Wood Protectors (Autodesk Fusion 360 design; units mm, degrees)
Autodesk Fusion 360 part; units mm, degrees
sketch "Sketch1" plane through (0, 0, 0) normal (0, 0, 1) x (1, 0, 0)
  circle A0 centre (-60, 0) radius 3
  circle A1 centre (-60, 0) radius 6.5
  dimension "d6" = 6
  dimension "d7" = 13
  constraint concentric A0 A1
  measures "d6" diameter of A0
  measures "d7" diameter of A1
sketch "Sketch2" plane through (0, 0, 0) normal (0, 0, 1) x (1, 0, 0)
  circle A0 centre (15.4632, 32.9185) radius 3
  circle A1 centre (9.4904, 74.3706) radius 3
  circle A2 centre (15.3555, 112.4631) radius 3
  line L0 (-7.5554, 127.9921) -> (32.4446, 127.9921)
  line L1 (32.4446, 127.9921) -> (32.4446, 17.9921)
  line L2 (32.4446, 17.9921) -> (-7.5554, 17.9921)
  line L3 (-7.5554, 17.9921) -> (-7.5554, 127.9921)
  dimension "d18" = 6
  dimension "d19" = 6
  dimension "d20" = 6
  dimension "d22" = 40
  dimension "d23" = 110
  constraint horizontal L0
  constraint vertical L1
  constraint horizontal L2
  constraint vertical L3
  measures "d18" diameter of A0
  measures "d19" diameter of A1
  measures "d20" diameter of A2
  measures "d22" distance of L1 L3
  measures "d23" distance of L0 L2
extrude "Extrude1" add sketch "Sketch1" along normal blind 1.5 contours A0 | A1
extrude "Extrude2" add sketch "Sketch1" against normal blind 3 contours A0
